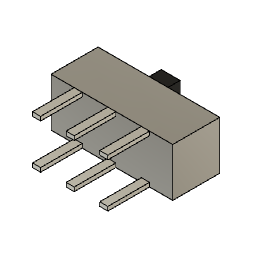
puntero34 (Autodesk Fusion 360 archive; units mm, degrees)
design "MSK-1153 slide switch"
Autodesk Fusion 360 part; units mm, degrees
sketch "Sketch1" plane through (0, 0, 0) normal (0, 0, 1) x (1, 0, 0)
  line L0 (-4.525, 3.5) -> (4.525, 3.5)
  line L1 (4.525, 3.5) -> (4.525, 0)
  line L2 (4.525, 0) -> (-4.525, 0)
  line L3 (-4.525, 0) -> (-4.525, 3.5)
  line L4 (-1.825, 5.5) -> (-0.425, 5.5)
  line L5 (-0.425, 5.5) -> (-0.425, 3.5)
  line L6 (-0.425, 3.5) -> (-1.825, 3.5)
  line L7 (-1.825, 3.5) -> (-1.825, 5.5)
  line L8 (-4.525, 0) -> (-4.525, -3.1) construction
  line L9 (-4.525, -3.1) -> (4.525, -3.1) construction
  line L10 (4.525, -3.1) -> (4.525, 0) construction
  line L11 (0, 0) -> (0, -3.1) construction
  line L12 (0.3, 0) -> (0.3, -3.1)
  line L13 (-0.3, -3.1) -> (-0.3, 0)
  line L14 (0.3, -1.55) -> (-0.3, -1.55) construction
  line L15 (-0.3, -3.1) -> (0.3, -3.1)
  line L16 (-2.8, 0) -> (-2.8, -3.1)
  line L17 (-2.2, -3.1) -> (-2.2, 0)
  line L18 (-2.5, 0) -> (-2.5, -3.1) construction
  line L19 (-2.8, -3.1) -> (-2.2, -3.1)
  line L20 (-2.8, -1.55) -> (-2.2, -1.55) construction
  line L21 (2.5, 0) -> (2.5, -3.1) construction
  line L22 (2.8, 0) -> (2.8, -3.1)
  line L23 (2.2, -3.1) -> (2.2, 0)
  line L24 (2.2, -1.55) -> (2.8, -1.55) construction
  line L25 (2.8, -3.1) -> (2.2, -3.1)
  line L26 (-2.025, 3.5) -> (-2.025, 2.9)
  line L27 (-2.025, 2.9) -> (2.025, 2.9)
  line L28 (2.025, 2.9) -> (2.025, 3.5)
  line L29 (-0.425, 5.5) -> (1.825, 5.5) construction
  line L30 (1.825, 5.5) -> (1.825, 3.5) construction
  dimension "d1" = 9.05
  dimension "d2" = 3.5
  dimension "d3" = 2
  dimension "d4" = 1.4
  dimension "d5" = 2.7
  dimension "d6" = 6.6
  dimension "d7" = 0.6
  dimension "d8" = 2.5
  dimension "d9" = 2.5
  dimension "d24" = 0.6
  dimension "d25" = 0.2
  dimension "d26" = 2.7
  dimension "d27" = 0.2
  constraint horizontal L0
  constraint vertical L1
  constraint horizontal L2
  constraint vertical L3
  constraint midpoint L11.start L2
  constraint horizontal L4
  constraint vertical L5
  constraint horizontal L6
  constraint vertical L7
  constraint coincident L0 L5.end
  constraint perpendicular L2 L8
  constraint perpendicular L1 L9
  constraint perpendicular L2 L10
  constraint coincident L11.start origin
  constraint midpoint L9 L11.end
  constraint coincident L2 L12.start
  constraint coincident L9 L12.end
  constraint coincident L9 L13.start
  constraint coincident L2 L13.end
  constraint vertical L13
  constraint vertical L12
  constraint midpoint L12 L14.start
  constraint midpoint L13 L14.end
  constraint midpoint L11 L14
  constraint coincident L2 L16.start
  constraint coincident L9 L16.end
  constraint coincident L9 L17.start
  constraint coincident L2 L17.end
  constraint vertical L17
  constraint vertical L16
  constraint coincident L2 L18.start
  constraint coincident L9 L18.end
  constraint perpendicular L9 L18
  constraint midpoint L16 L20.start
  constraint midpoint L17 L20.end
  constraint equal L14 L20
  constraint midpoint L18 L20
  constraint coincident L2 L21.start
  constraint coincident L9 L21.end
  constraint perpendicular L9 L21
  constraint coincident L2 L22.start
  constraint coincident L9 L22.end
  constraint coincident L9 L23.start
  constraint coincident L2 L23.end
  constraint vertical L23
  constraint vertical L22
  constraint midpoint L23 L24.start
  constraint midpoint L22 L24.end
  constraint midpoint L21 L24
  constraint equal L14 L24
  constraint coincident L0 L26.start
  constraint perpendicular L0 L26
  constraint perpendicular L26 L27
  constraint coincident L0 L28.end
  constraint perpendicular L0 L28
  constraint perpendicular L5 L29
  constraint coincident L0 L30.end
  constraint perpendicular L0 L30
  measures "d1" distance of L0.start L0.end
  measures "d2" distance of L0.start L2.end
  measures "d3" distance of L4 L6
  measures "d4" distance of L5 L7
  measures "d5" distance of L0.start L7
  measures "d6" distance of L0 L9
  measures "d7" distance of L14.start L14.end
  measures "d8" distance of L11 L18
  measures "d9" distance of L11 L21
  measures "d24" distance of L0 L27
  measures "d25" distance of L7 L26
  measures "d26" distance of L0.end L30
  measures "d27" distance of L28 L30
extrude "Extrude2" add sketch "Sketch1" along normal blind 1.8 and the other way blind 1.8 contours L0 L1 L2 L3 L26 L27 L28 | L0 L6 L26 L27 L28 makes body 1
extrude "Extrude1" add sketch "Sketch1" against normal blind 0.3 from surface at 1.8 separate body contours L2 L16 L17 L19 | L2 L12 L13 L15 | L2 L22 L23 L25 makes body 2 at (-2.6, -1.0333, 1.8) makes body 3 at (-0.1, -1.0333, 1.8) makes body 4 at (2.4, -1.0333, 1.8)
extrude "Extrude3" add sketch "Sketch1" along normal blind 0.3 from surface at -1.8 separate body contours L2 L16 L17 L19 | L2 L12 L13 L15 | L2 L22 L23 L25 makes body 5 at (-2.6, -1.0333, -1.8) makes body 6 at (-0.1, -1.0333, -1.8) makes body 7 at (2.4, -1.0333, -1.8)
extrude "Extrude4" add sketch "Sketch1" along normal blind 0.7 and the other way blind 0.7 separate body contours L0 L4 L5 L6 L7 makes body 8
extrude "Extrude5" add sketch "Sketch1" along normal up to surface (0.9 mm away) and the other way up to surface (0.9 mm away) separate body contours L0 L6 L26 L27 L28 makes body 9
combine "Combine1" operation cut target body 1 tool bodies 9 keep tools
move_body "Move1" bodies 9 to x (1, 0, 0) y (0, 1, 0) z (0, 0, 1) at (0, -0.2, 0)
extrude "Extrude6" add 1 faces at (-1.3583, 3.5, -0.2333) along direction (0, -1, 0) blind 0.5 on bodies 8 bodies 8 9

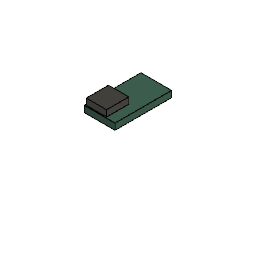
design "pat9125el-breakout"
Autodesk Fusion 360 part; units mm, degrees
ref_plane "WorkPlane1" through (0, 0, -2) normal (0, 0, 1) x (1, 0, 0)
sketch "top" plane through (0, 0, -2) normal (0, 0, 1) x (1, 0, 0)
  line L0 (-1.75, 6.99) -> (3.075, 6.99)
  line L1 (3.075, 6.99) -> (3.075, -1.91)
  line L2 (3.075, -1.91) -> (-1.75, -1.91)
  line L3 (-1.75, -1.91) -> (-1.75, 6.99)
  line L4 (-1.6, 1.74) -> (1.6, 1.74)
  line L5 (1.6, 1.74) -> (1.6, -1.76)
  line L6 (1.6, -1.76) -> (-1.6, -1.76)
  line L7 (-1.6, -1.76) -> (-1.6, 1.74)
  line L8 (0, 0) -> (0, 1.74) construction
  dimension "d1" = 8.9
  dimension "d2" = 4.825
  dimension "d3" = 3.5
  dimension "d4" = 3.2
  dimension "d21" = 0.15
  dimension "d22" = 0.15
  dimension "d23" = 1.74
  constraint horizontal L0
  constraint vertical L1
  constraint horizontal L2
  constraint vertical L3
  constraint horizontal L4
  constraint vertical L5
  constraint horizontal L6
  constraint vertical L7
  constraint midpoint L4 L8.end
  constraint perpendicular L4 L8
  constraint coincident L8.start origin
  measures "d1" distance of L0.start L2.end
  measures "d2" distance of L0.start L0.end
  measures "d3" distance of L4.start L6.end
  measures "d4" distance of L4.start L4.end
  measures "d21" distance of L2 L6
  measures "d22" distance of L3 L7
  measures "d23" distance of L8.start L8.end
extrude "Extrude3" add sketch "top" against normal blind 1 contours L0 L1 L2 L3 | L4 L5 L6 L7 makes body 1
ref_plane "WorkPlane2" through (0, 0, -1) normal (0, 0, 1) x (1, 0, 0)
extrude "Extrude4" add sketch "top" along normal up to surface (0.99 mm away) from surface at 0.01 separate body contours L4 L5 L6 L7 makes body 2

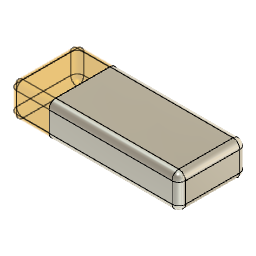
design "Lipo 200mAh 601230"
Autodesk Fusion 360 part; units mm, degrees
sketch "Sketch1" plane through (0, 0, 0) normal (0, 0, 1) x (1, 0, 0) in component "Lipo_Body"
  line L0 (15, -6) -> (-15, -6)
  line L1 (-15, -6) -> (-15, 6)
  line L2 (-15, 6) -> (15, 6)
  line L3 (15, 6) -> (15, -6)
  line L4 (15, -6) -> (-15, 6) construction
  line L5 (-15, -6) -> (15, 6) construction
  line L6 (-8, 6) -> (-8, -6)
  dimension "d1" = 30
  dimension "d3" = 7
  dimension "d74" = 12
  constraint horizontal L0
  constraint perpendicular L0 L1
  constraint parallel L0 L2
  constraint parallel L1 L3
  constraint coincident L4 origin
  constraint coincident L5 origin
  constraint coincident L2 L6.start
  constraint coincident L0 L6.end
  constraint perpendicular L0 L6
  measures "d1" distance of L1.end L2.end
  measures "d3" distance of L1 L6
  measures "d74" distance of L0 L2
extrude "Extrude1" add sketch "Sketch1" along normal blind 6 contours L0 L2 L3 L6 makes body 1 in component "Lipo_Body"
extrude "Extrude2" add sketch "Sketch1" along normal up to surface (6 mm away) separate body contours L0 L1 L2 L6 makes body 2 in component "Lipo_Body"
fillet "Fillet1" radius 1.2 16 edges at (15, -6, 3) (15, 6, 3) (15, 0, 0) (15, 0, 6) (3.5, -6, 6) (3.5, -6, 0) (3.5, 6, 6) (3.5, 6, 0) (-15, -6, 3) (-15, 6, 3) (-15, 0, 6) (-15, 0, 0) (-11.5, -6, 6) (-11.5, -6, 0) (-11.5, 6, 6) (-11.5, 6, 0) on bodies 1 2 in component "Lipo_Body"
shell "Shell2" thickness 0.1 removed faces 0 bodies 2 in component "Lipo_Body"
component "Lipo_Body" placed x (1, 0, 0) y (0, 1, 0) z (0, 0, 1) at (0, 0, 0)
equation "d5_1 = 0.1 mm + 0.05 mm"
equation "d9_1 = 0.1 mm - 0.05 mm"
equation "d13_1 = ( 2.8 / 2 ) * 1 mm"
equation "d19_1 = ( 1.9 / 2 ) * 1 mm"
equation "d20_1 = ( -1.9 / 2 ) * 1 mm"
equation "d13_2 = ( 2.8 / 2 ) * 1 mm"
equation "d19_2 = ( 1.9 / 2 ) * 1 mm"
equation "d20_2 = ( -1.9 / 2 ) * 1 mm"
equation "d80 = 1.6 mm - 0.3 mm"
named bodies: "sticker"
